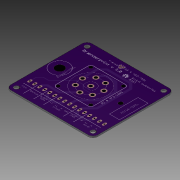
# Autodesk Inventor part: pcb-model
Saved by Autodesk Inventor 2015 (Build 190159000, 159)
## iProperties
Created: 2013-08-12
Part Number: pcb-model
Material: Generic
Document SubType Name: Modeling
Designer: stoffer
Density: 1 g/cm^3
Appearance: Default
Mass: 10.8382 g
Surface Area: 150.363 cm^2
Volume: 10.8382 cm^3
Author: stoffer
Autodesk Inventor part; units mm, degrees
ref_plane "YZ Plane" through (0, 0, 0) normal (1, 0, 0) x (0, 1, 0)
ref_plane "XZ Plane" through (0, 0, 0) normal (0, 1, 0) x (-1, 0, 0)
ref_plane "XY Plane" through (0, 0, 0) normal (0, 0, 1) x (1, 0, 0)
sketch "Sketch1" plane through (0, 0, 0) normal (0, 0, 1) x (1, 0, 0)
  line L0 (5, 0) -> (83.57, 0)
  line L1 (88.57, 5) -> (88.57, 77.54)
  line L2 (83.57, 82.54) -> (5, 82.54)
  line L3 (0, 77.54) -> (0, 5)
  line L4 (5.285, 77.27) -> (83.285, 77.27) construction
  line L5 (83.285, 77.27) -> (83.285, 5.27) construction
  line L6 (83.285, 5.27) -> (5.285, 5.27) construction
  line L7 (5.285, 5.27) -> (5.285, 77.27) construction
  arc A0 (5, 82.54) -> (0, 77.54) centre (5, 77.54) ccw
  arc A1 (0, 5) -> (5, 0) centre (5, 5) ccw
  arc A2 (83.57, 0) -> (88.57, 5) centre (83.57, 5) ccw
  arc A3 (88.57, 77.54) -> (83.57, 82.54) centre (83.57, 77.54) ccw
  circle A4 centre (5.285, 77.27) radius 2.25
  circle A5 centre (83.285, 77.27) radius 2.25
  circle A6 centre (83.285, 5.27) radius 2.25
  circle A7 centre (5.285, 5.27) radius 2.25
  point P0 (0, 0)
  point P1 (88.57, 82.54)
  point P2 (0, 82.54)
  dimension "d0" = 88.57
  dimension "d2" = 82.54
  dimension "d3" = 78
  dimension "d4" = 72
  dimension "d5" = 5.285
  dimension "d6" = 5.27
  dimension "d7" = 5
  dimension "d8" = 4.5
  dimension "d9" = 4.5
  dimension "d10" = 4.5
  dimension "d11" = 4.5
  constraints: 16 end point, 8 centre point, 8 coincident, 8 point on circle, 8 tangent, 6 point on line, 4 parallel, 3 equal radius, 2 horizontal, 2 perpendicular
  measures "d0" distance of point (88.57, 82.54) point (0, 82.54)
  measures "d2" distance of point (0, 82.54) point (0, 0)
  measures "d3" distance of L4.start L4.end
  measures "d4" distance of L6.end L4.start
  measures "d5" distance between parallel lines of L7 L3
  measures "d6" distance between parallel lines of L0 L6
  measures "d7" radius of A0
  measures "d8" diameter of A4
  measures "d9" diameter of A5
  measures "d10" diameter of A6
  measures "d11" diameter of A7
extrude "Extrusion1" add sketch "Sketch1" along normal blind 1.5
sketch "Sketch2" plane through (0, 0, 1.5) normal (0, 0, 1) x (1, 0, 0)
  line L0 (0, 77.54) -> (0, 5) projected
  line L1 (88.57, 5) -> (88.57, 77.54) projected
  line L2 (83.57, 82.54) -> (5, 82.54) projected
  line L3 (0, 82.54) -> (88.57, 82.54) construction
  line L4 (88.57, 82.54) -> (88.57, -0.0156) construction
  line L5 (88.57, -0.0156) -> (0, -0.0156) construction
  line L6 (0, -0.0156) -> (0, 82.54) construction
  point P0 (0, 0)
  constraints: 3 collinear, 2 other
decal "Decal1"
sketch "Sketch3" plane through (0, 0, 0) normal (0, 0, -1) x (-1, 0, 0)
  line L0 (0, 77.54) -> (0, 5) projected
  line L1 (-83.57, 82.54) -> (-5, 82.54) projected
  line L2 (-88.57, 5) -> (-88.57, 77.54) projected
  line L3 (-88.57, 82.54) -> (0, 82.54) construction
  line L4 (0, 82.54) -> (0, -0.0156) construction
  line L5 (0, -0.0156) -> (-88.57, -0.0156) construction
  line L6 (-88.57, -0.0156) -> (-88.57, 82.54) construction
  point P0 (0, 0)
  constraints: 3 collinear, 2 other
decal "Decal2"
equation "\"d5\" = -0.5 * d3 + 0.5 * d0"
equation "\"d6\" = -0.5 * d4 + 0.5 * d2"
equation "\"d9\" = d8"
equation "\"d10\" = d8"
equation "\"d11\" = d8"
body "Solid1"
